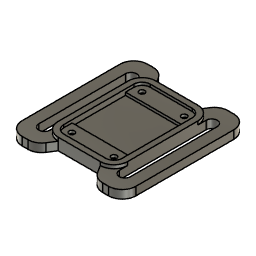
SquidSlimeCaseAUX (Autodesk Fusion 360 design; units mm, degrees)
Autodesk Fusion 360 part; units mm, degrees
note: some values were not read from the file. Set by a fixed rule: which face or edge a step refers to.
sketch "スケッチ1" plane through (0, 0, 0) normal (0, 0, 1) x (1, 0, 0)
  line L0 (52.54, 69.52) -> (67.78, 69.52)
  line L1 (70.32, 72.06) -> (70.32, 97.46)
  line L2 (67.78, 100) -> (52.54, 100)
  line L3 (50, 97.46) -> (50, 72.06)
  arc A0 (52.54, 100) -> (50, 97.46) centre (52.54, 97.46) ccw
  arc A1 (70.32, 97.46) -> (67.78, 100) centre (67.78, 97.46) ccw
  arc A2 (67.78, 69.52) -> (70.32, 72.06) centre (67.78, 72.06) ccw
  arc A3 (50, 72.06) -> (52.54, 69.52) centre (52.54, 72.06) ccw
  circle A4 centre (52.54, 97.46) radius 1
  circle A5 centre (67.78, 97.46) radius 1
  circle A6 centre (67.78, 72.06) radius 1
  circle A7 centre (52.54, 72.06) radius 1
  line L4 (60.16, 92.4) -> (60.16, 77.12)
  line L5 (65.24, 92.4) -> (55.08, 92.4)
  line L6 (55.08, 77.12) -> (65.24, 77.12)
  line L7 (55.08, 100) -> (55.08, 92.4)
  line L8 (55.08, 77.12) -> (55.08, 69.52)
  line L9 (65.24, 100) -> (65.24, 92.4)
  line L10 (65.24, 77.12) -> (65.24, 69.52)
  dimension "d7" = 2.54
  dimension "d8" = 2
  dimension "d9" = 2
  dimension "d10" = 2
  dimension "d11" = 2
  constraint horizontal L0
  constraint vertical L1
  constraint horizontal L2
  constraint vertical L3
  constraint tangent L2 A0
  constraint tangent L3 A0
  constraint tangent L1 A1
  constraint tangent L2 A1
  constraint equal A0 A1
  constraint tangent L0 A2
  constraint tangent L1 A2
  constraint equal A0 A2
  constraint tangent L3 A3
  constraint tangent L0 A3
  constraint equal A0 A3
  constraint concentric A0 A4
  constraint concentric A1 A5
  constraint concentric A2 A6
  constraint concentric A3 A7
  constraint coincident L6.start L7
  constraint collinear L7 L8
  constraint coincident L6 L4.end
  constraint coincident L6.end L9
  constraint collinear L9 L10
  constraint coincident L5 L4.start
  measures "d7" radius of A0
  measures "d8" diameter of A4
  measures "d9" diameter of A5
  measures "d10" diameter of A6
  measures "d11" diameter of A7
extrude "押し出し1" add sketch "スケッチ1" along normal blind 4.8 contours L0 L6 L8 L10 | L2 L5 L7 L9 makes body 1 at (61.8533, 94.9333, 0) makes body 2 at (58.4667, 72.0533, 0)
extrude "押し出し2" add 1 faces at (58.4667, 69.52, 3.2) along direction (0, -1, 0) blind 0.1 on bodies 2 bodies 2
extrude "押し出し3" add 1 faces at (61.8533, 100, 3.2) along direction (0, 1, 0) blind 0.1 on bodies 1 bodies 1
extrude "押し出し4" add sketch "スケッチ1" against normal blind 1 separate body makes body 3
combine "結合1" operation add target body 3 tool bodies 1 2
sketch "スケッチ2" plane through (0, 0, -1) normal (0, 0, -1) x (1, 0, 0)
  circle A0 centre (67.78, -72.06) radius 1
  circle A1 centre (52.54, -72.06) radius 1
  circle A2 centre (67.78, -97.46) radius 1
  circle A3 centre (52.54, -97.46) radius 1
  arc A4 (52.54, -69.52) -> (50, -72.06) centre (52.54, -72.06) ccw
  line L0 (50, -72.06) -> (50, -97.46)
  arc A5 (50, -97.46) -> (52.54, -100) centre (52.54, -97.46) ccw
  line L1 (52.54, -100) -> (67.78, -100)
  arc A6 (67.78, -100) -> (70.32, -97.46) centre (67.78, -97.46) ccw
  line L2 (70.32, -97.46) -> (70.32, -72.06)
  arc A7 (70.32, -72.06) -> (67.78, -69.52) centre (67.78, -72.06) ccw
  line L3 (67.78, -69.52) -> (52.54, -69.52)
  line L4 (52.54, -100.4) -> (67.78, -100.4)
  arc A8 (67.78, -100.4) -> (70.72, -97.46) centre (67.78, -97.46) ccw
  line L5 (70.72, -97.46) -> (70.72, -72.06)
  arc A9 (70.72, -72.06) -> (67.78, -69.12) centre (67.78, -72.06) ccw
  line L6 (67.78, -69.12) -> (52.54, -69.12)
  arc A10 (52.54, -69.12) -> (49.6, -72.06) centre (52.54, -72.06) ccw
  line L7 (49.6, -72.06) -> (49.6, -97.46)
  arc A11 (49.6, -97.46) -> (52.54, -100.4) centre (52.54, -97.46) ccw
  line L8 (52.54, -102.4) -> (67.78, -102.4)
  arc A12 (67.78, -102.4) -> (72.72, -97.46) centre (67.78, -97.46) ccw
  line L9 (72.72, -97.46) -> (72.72, -72.06)
  arc A13 (72.72, -72.06) -> (67.78, -67.12) centre (67.78, -72.06) ccw
  line L10 (67.78, -67.12) -> (52.54, -67.12)
  arc A14 (52.54, -67.12) -> (47.6, -72.06) centre (52.54, -72.06) ccw
  line L11 (47.6, -72.06) -> (47.6, -97.46)
  arc A15 (47.6, -97.46) -> (52.54, -102.4) centre (52.54, -97.46) ccw
  line L12 (60.16, -67.12) -> (60.16, -102.4)
  line L13 (55.08, -67.12) -> (55.08, -102.4)
  line L14 (65.24, -67.12) -> (65.24, -102.4)
  dimension "d24" = 0.4
  dimension "d25" = 2.4
  dimension "d58" = 5.08
  dimension "d59" = -5.08
  constraint midpoint L10 L12.start
  constraint midpoint L8 L12.end
extrude "押し出し5" add sketch "スケッチ2" against normal blind 1 separate body contours L6 L10 L12 L13 | L4 L6 A10 L7 A11 L8 L10 A14 L11 A15 L13 | L6 L10 L12 L14 | L4 L8 L12 L13 | L4 A8 L5 A9 L6 L8 A12 L9 A13 L10 L14 | L4 L8 L12 L14 makes body 4
extrude "押し出し6" add sketch "スケッチ2" along normal blind 1 bodies 4
extrude "押し出し7" add sketch "スケッチ2" along normal blind 1 contours A0 | A1 | A2 | A3 bodies 4
extrude "押し出し8" add sketch "スケッチ2" against normal blind 8 separate body contours A0 | A1 | A2 | A3 | A4 L0 A5 L1 L3 L13 | A4 L0 A5 L1 L3 L4 L6 A10 L7 A11 L13 | L3 L6 L12 L13 | L1 L3 L12 L13 | L3 L6 L12 L14 | L1 L3 L12 L14 | L6 L10 L12 L13 | L4 L6 A10 L7 A11 L8 L10 A14 L11 A15 L13 | L1 L4 L12 L13 | L1 A6 L2 A7 L3 L4 A8 L5 A9 L6 L14 | L1 A6 L2 A7 L3 L14 | L6 L10 L12 L14 | L1 L4 L12 L14 | L4 L8 L12 L13 | L4 A8 L5 A9 L6 L8 A12 L9 A13 L10 L14 | L4 L8 L12 L14 makes body 5
extrude "押し出し9" cut 1 faces at (64.3467, 88.9933, -1) along direction (0, 0, 1) blind 1 on bodies 5 bodies 5
extrude "押し出し10" cut 2 faces at (61.8533, 94.9667, 4.8) (58.4667, 71.9867, 4.8) along direction (0, 0, 1) blind 7 on bodies 3 bodies 5
extrude "押し出し11" cut 1 faces at (58.4667, 69.42, 5.5333) along direction (0, -1, 0) blind 10 on bodies 5 bodies 5
extrude "押し出し12" cut 1 faces at (61.8533, 100.1, 5.5333) along direction (0, 1, 0) blind 11 on bodies 5 bodies 5
extrude "押し出し13" cut 1 faces at (61.8533, 100.1, 3.2) along direction (0, 1, 0) blind 8 on bodies 3 bodies 5
extrude "押し出し14" cut 1 faces at (58.4667, 69.42, 3.2) along direction (0, -1, 0) blind 9 on bodies 3 bodies 5
extrude "押し出し15" cut sketch "スケッチ2" against normal blind 5.8 contours A0 | A1 | A2 | A3 | A4 L0 A5 L1 L3 L13 | A4 L0 A5 L1 L3 L4 L6 A10 L7 A11 L13 | L3 L6 L12 L13 | L1 L3 L12 L13 | L3 L6 L12 L14 | L1 L3 L12 L14 | L1 L4 L12 L13 | L1 A6 L2 A7 L3 L4 A8 L5 A9 L6 L14 | L1 A6 L2 A7 L3 L14 | L1 L4 L12 L14 bodies 5
extrude "押し出し16" cut 2 faces at (65.24, 98.4, 6.2667) (65.24, 71.12, 6.2667) along direction (1, 0, 0) blind 0.25 on bodies 5 bodies 5
extrude "押し出し17" cut 2 faces at (55.08, 71.12, 6.2667) (55.08, 98.4, 6.2667) along direction (-1, 0, 0) blind 0.25 on bodies 5 bodies 5
extrude "押し出し18" cut 1 faces at (61.9367, 92.4, 6.2667) along direction (0, -1, 0) blind 0.25 on bodies 5 bodies 5
extrude "押し出し19" cut 1 faces at (61.9367, 77.12, 5.5333) along direction (0, 1, 0) blind 0.25 on bodies 5 bodies 5
extrude "押し出し20" cut sketch "スケッチ1" against normal blind 12 contours A4 | A5 | A6 | A7 bodies 4
extrude "押し出し21" add sketch "スケッチ2" against normal blind 5.8 contours A4 L0 A5 L1 L3 L13 | A4 L0 A5 L1 L3 L4 L6 A10 L7 A11 L13 | L1 A6 L2 A7 L3 L4 A8 L5 A9 L6 L14 | L1 A6 L2 A7 L3 L14 bodies 5
extrude "押し出し22" cut 2 faces at (69.8618, 88.683, -1) (50.4582, 88.683, -1) along direction (0, 0, 1) blind 1 on bodies 5 bodies 5
extrude "押し出し23" cut 1 faces at (65.24, 82.2967, 1.6) along direction (1, 0, 0) blind 0.25 on bodies 5 bodies 5
extrude "押し出し24" cut 1 faces at (55.08, 82.2967, 1.6) along direction (-1, 0, 0) blind 0.25 on bodies 5 bodies 5
extrude "押し出し25" cut 1 faces at (58.3833, 87.2233, 7) along direction (0, 0, -1) blind 0.2 on bodies 5 bodies 5
extrude "押し出し26" add 1 faces at (57.7867, 88.7047, -2) along direction (0, 0, -1) blind 1.5 separate body on bodies 4 makes body 6
move_face "面をオフセット1" offset -0.75 4 faces at (51.8783, 71.3102, -3) (53.5091, 97.7068, -3) (67.014, 96.8172, -3) (68.7491, 72.3068, -3) on bodies 6
combine "結合2" operation add target body 4 tool bodies 6
extrude "押し出し27" add 1 faces at (57.9117, 88.4882, -3.5) along direction (0, 0, -1) blind 0.5 on bodies 4 bodies 4
sketch "スケッチ3" plane through (0, 0, -4) normal (0, 0, -1) x (1, 0, 0)
  circle A0 centre (52.54, -97.46) radius 1.75
  circle A1 centre (52.54, -72.06) radius 1.75
  circle A2 centre (67.78, -97.46) radius 1.75
  circle A3 centre (67.78, -72.06) radius 1.75
  arc A4 (47.6, -97.46) -> (52.54, -102.4) centre (52.54, -97.46) ccw
  line L0 (52.54, -102.4) -> (67.78, -102.4)
  arc A5 (67.78, -102.4) -> (72.72, -97.46) centre (67.78, -97.46) ccw
  line L1 (72.72, -97.46) -> (72.72, -72.06)
  arc A6 (72.72, -72.06) -> (67.78, -67.12) centre (67.78, -72.06) ccw
  line L2 (67.78, -67.12) -> (52.54, -67.12)
  arc A7 (52.54, -67.12) -> (47.6, -72.06) centre (52.54, -72.06) ccw
  line L3 (47.6, -72.06) -> (47.6, -97.46)
  line L4 (76.72, -97.46) -> (76.72, -74.06)
  line L5 (80.72, -97.46) -> (80.72, -72.06)
  line L6 (43.6, -74.06) -> (43.6, -97.46)
  line L7 (39.6, -72.06) -> (39.6, -97.46)
  line L8 (60.16, -67.12) -> (60.16, -102.4)
  arc A8 (80.72, -72.06) -> (75.78, -67.12) centre (75.78, -72.06) ccw
  arc A9 (44.54, -67.12) -> (39.6, -72.06) centre (44.54, -72.06) ccw
  line L9 (44.54, -67.12) -> (75.78, -67.12)
  line L10 (47.6, -84.76) -> (72.72, -84.76)
  line L11 (47.6, -74.06) -> (47.6, -97.46)
  line L12 (72.72, -74.06) -> (72.72, -97.46)
  arc A10 (45.6, -72.06) -> (43.6, -74.06) centre (45.6, -74.06) ccw
  arc A11 (47.6, -74.06) -> (45.6, -72.06) centre (45.6, -74.06) ccw
  arc A12 (74.72, -72.06) -> (72.72, -74.06) centre (74.72, -74.06) ccw
  arc A13 (76.72, -74.06) -> (74.72, -72.06) centre (74.72, -74.06) ccw
  arc A14 (75.78, -102.4) -> (80.72, -97.46) centre (75.78, -97.46) ccw
  arc A15 (74.72, -97.46) -> (76.72, -95.46) centre (74.72, -95.46) ccw
  arc A16 (72.72, -95.46) -> (74.72, -97.46) centre (74.72, -95.46) ccw
  line L13 (44.54, -102.4) -> (75.78, -102.4)
  arc A17 (39.6, -97.46) -> (44.54, -102.4) centre (44.54, -97.46) ccw
  arc A18 (43.6, -95.46) -> (45.6, -97.46) centre (45.6, -95.46) ccw
  arc A19 (45.6, -97.46) -> (47.6, -95.46) centre (45.6, -95.46) ccw
  dimension "d76" = 8
  dimension "d78" = 8
  dimension "d79" = 2
  constraint midpoint L2 L8.start
  constraint midpoint L0 L8.end
  constraint symmetric L8 L5.end L7.start
  constraint symmetric L8 A8.end A9.start
  constraint symmetric L8 A8 A9
  constraint tangent A8 L9
  constraint midpoint L3 L10.start
  constraint midpoint L1 L10.end
  constraint coincident A4.start L3.end
  constraint coincident A5.end L1.start
  constraint tangent L6 A10
  constraint tangent L11 A11
  constraint equal A10 A11
  constraint coincident A10.start A11.end
  constraint tangent L12 A12
  constraint equal A10 A12
  constraint tangent L4 A13
  constraint equal A10 A13
  constraint coincident A12.start A13.end
  constraint symmetric L5.end L10 L5.start
  constraint symmetric A8.end L10 A14.start
  constraint symmetric A8 L10 A14
  constraint symmetric L7.start L10 L7.end
  constraint symmetric A9.start L10 L13.start
  constraint symmetric A9 L10 A17
  constraint symmetric L10 L6.start A18.start
  constraint symmetric L10 A10.start A18.end
  constraint symmetric L10 A10 A18
  constraint symmetric L10 L11.start A19.end
  constraint symmetric L10 A11 A19
  constraint symmetric L10 A12.start A15.start
  constraint symmetric L10 L12.start A16.start
  constraint symmetric L10 A12 A16
  constraint symmetric L10 L4.end A15.end
  constraint symmetric L10 A13 A15
  measures "d79" radius of A10
extrude "押し出し28" add sketch "スケッチ3" against normal blind 4 separate body contours A4 A7 L3 L6 L7 A9 L9 L11 A10 A11 L13 A17 A18 A19 | A5 L1 A6 L4 L5 A8 L9 L12 A12 A13 A14 A15 A16 L13 makes body 7 at (40.9333, 81.1933, 0) makes body 8 at (79.3867, 88.3267, -4)
combine "結合3" operation add target body 4 tool bodies 7 8
extrude "押し出し29" cut sketch "スケッチ3" against normal blind 12 contours A4 A7 L3 L6 L7 A9 L9 L11 A10 A11 L13 A17 A18 A19 | A5 L1 A6 L4 L5 A8 L9 L12 A12 A13 A14 A15 A16 L13 bodies 4
extrude "押し出し30" add sketch "スケッチ3" against normal blind 3 contours A4 A7 L3 L6 L7 A9 L9 L11 A10 A11 L13 A17 A18 A19 | A5 L1 A6 L4 L5 A8 L9 L12 A12 A13 A14 A15 A16 L13 bodies 4
copy_body "ボディのコピーと貼り付け1" bodies 4 makes body 9
extrude "押し出し31" cut 2 faces at (40.9333, 81.1933, -1) (79.3867, 88.3267, -1) along direction (0, 0, -1) blind 12 on bodies 9 bodies 9
sketch "スケッチ4" plane through (0, 0, -4) normal (0, 0, -1) x (1, 0, 0)
  arc A0 (75.78, -117.4) -> (80.72, -112.46) centre (75.78, -112.46) ccw
  arc A1 (74.72, -112.46) -> (76.72, -110.46) centre (74.72, -110.46) ccw
  arc A2 (72.72, -110.46) -> (74.72, -112.46) centre (74.72, -110.46) ccw
  arc A3 (68.72, -112.46) -> (73.66, -117.4) centre (73.66, -112.46) ccw
  line L0 (75.78, -117.4) -> (73.66, -117.4)
  line L1 (47.6, -84.76) -> (72.72, -84.76)
  arc A4 (80.72, -57.06) -> (75.78, -52.12) centre (75.78, -57.06) ccw
  arc A5 (73.66, -52.12) -> (68.72, -57.06) centre (73.66, -57.06) ccw
  arc A6 (76.72, -59.06) -> (74.72, -57.06) centre (74.72, -59.06) ccw
  line L2 (75.78, -52.12) -> (73.66, -52.12)
  arc A7 (74.72, -57.06) -> (72.72, -59.06) centre (74.72, -59.06) ccw
  line L3 (80.72, -112.46) -> (80.72, -57.06)
  arc A8 (72.72, -72.06) -> (67.78, -67.12) centre (67.78, -72.06) ccw
  line L4 (68.72, -57.06) -> (67.78, -67.12)
  arc A9 (67.78, -102.4) -> (72.72, -97.46) centre (67.78, -97.46) ccw
  line L5 (68.72, -112.46) -> (67.78, -102.4)
  line L6 (76.72, -59.06) -> (76.72, -110.46)
  line L7 (72.72, -59.06) -> (72.72, -110.46)
  line L8 (60.16, -67.12) -> (60.16, -102.4)
  line L9 (43.6, -59.06) -> (43.6, -110.46)
  arc A10 (46.66, -117.4) -> (51.6, -112.46) centre (46.66, -112.46) ccw
  line L10 (44.54, -117.4) -> (46.66, -117.4)
  arc A11 (45.6, -112.46) -> (47.6, -110.46) centre (45.6, -110.46) ccw
  arc A12 (43.6, -110.46) -> (45.6, -112.46) centre (45.6, -110.46) ccw
  line L11 (47.6, -59.06) -> (47.6, -110.46)
  arc A13 (45.6, -57.06) -> (43.6, -59.06) centre (45.6, -59.06) ccw
  line L12 (39.6, -112.46) -> (39.6, -57.06)
  arc A14 (52.54, -67.12) -> (47.6, -72.06) centre (52.54, -72.06) ccw
  line L13 (51.6, -57.06) -> (52.54, -67.12)
  arc A15 (39.6, -112.46) -> (44.54, -117.4) centre (44.54, -112.46) ccw
  arc A16 (47.6, -97.46) -> (52.54, -102.4) centre (52.54, -97.46) ccw
  arc A17 (47.6, -59.06) -> (45.6, -57.06) centre (45.6, -59.06) ccw
  arc A18 (44.54, -52.12) -> (39.6, -57.06) centre (44.54, -57.06) ccw
  line L14 (44.54, -52.12) -> (46.66, -52.12)
  arc A19 (51.6, -57.06) -> (46.66, -52.12) centre (46.66, -57.06) ccw
  line L15 (51.6, -112.46) -> (52.54, -102.4)
  point P0 (47.6, -84.76)
  constraint tangent A3 L0
  constraint symmetric A0.start L1 A4.end
  constraint symmetric A0.end L1 A4.start
  constraint symmetric A0 L1 A4
  constraint symmetric A2.start L1 A7.end
  constraint symmetric A1.start L1 A6.end
  constraint symmetric A1.end L1 A6.start
  constraint symmetric A1 L1 A6
  constraint symmetric A2 L1 A7
  constraint symmetric A3.end L1 A5.start
  constraint symmetric A3.start L1 A5.end
  constraint symmetric A3 L1 A5
  constraint tangent A4 L3
  constraint symmetric L1 A5.end A3.start
  constraint symmetric L1 A8.start A9.end
  constraint symmetric L1 A8.end A9.start
  constraint symmetric L1 A8 A9
  constraint tangent A1 L6
  constraint tangent A2 L7
  constraint symmetric A0.start L8 L10.start
  constraint symmetric A0.end L8 L12.start
  constraint symmetric A0 L8 A15
  constraint symmetric A2.start L8 A11.end
  constraint symmetric A1.start L8 A11.start
  constraint symmetric A1.end L8 L9.end
  constraint symmetric A1 L8 A12
  constraint symmetric A2 L8 A11
  constraint symmetric A3.end L8 A10.start
  constraint symmetric A3.start L8 A10.end
  constraint symmetric A3 L8 A10
  constraint symmetric L1.end L8 P0
  constraint symmetric A7.end L8 L11.start
  constraint symmetric A6.start L8 L9.start
  constraint symmetric A5.start L8 L14.end
  constraint symmetric A4.start L8 L12.end
  constraint symmetric A4.end L8 A18.start
  constraint symmetric A6.end L8 A13.start
  constraint symmetric A5.end L8 L13.start
  constraint symmetric A4 L8 A18
  constraint symmetric A5 L8 A19
  constraint symmetric A6 L8 A13
  constraint symmetric A7 L8 A17
  constraint symmetric A8.start L8 A14.end
  constraint symmetric A8.end L8 A14.start
  constraint symmetric A8 L8 A14
  constraint symmetric A9.end L8 A16.start
  constraint symmetric A9.start L8 A16.end
  constraint symmetric A9 L8 A16
extrude "押し出し32" add sketch "スケッチ4" against normal blind 3 contours A0 A1 A2 A3 L0 A4 A5 A6 L2 A7 L3 A8 L4 A9 L5 L6 L7 | L9 A10 L10 A11 A12 L11 A13 L12 A14 L13 A15 A16 A17 A18 L14 A19 L15 bodies 9
sketch "スケッチ5" plane through (0, 0, -1) normal (0, 0, 1) x (-1, 0, 0)
  circle A0 centre (-52.54, -97.46) radius 1
  circle A1 centre (-52.54, -72.06) radius 1
  circle A2 centre (-67.78, -97.46) radius 1
  circle A3 centre (-67.78, -72.06) radius 1
  line L0 (-49.6, -97.46) -> (-49.6, -72.06)
  arc A4 (-49.6, -72.06) -> (-52.54, -69.12) centre (-52.54, -72.06) ccw
  line L1 (-52.54, -69.12) -> (-67.78, -69.12)
  arc A5 (-67.78, -69.12) -> (-70.72, -72.06) centre (-67.78, -72.06) ccw
  line L2 (-70.72, -72.06) -> (-70.72, -97.46)
  arc A6 (-70.72, -97.46) -> (-67.78, -100.4) centre (-67.78, -97.46) ccw
  line L3 (-67.78, -100.4) -> (-52.54, -100.4)
  arc A7 (-52.54, -100.4) -> (-49.6, -97.46) centre (-52.54, -97.46) ccw
  line L4 (-60.16, -75.12) -> (-49.6, -75.12)
  line L5 (-60.16, -75.12) -> (-70.72, -75.12)
  line L6 (-49.6, -84.76) -> (-70.72, -84.76)
  line L7 (-60.16, -94.4) -> (-49.6, -94.4)
  line L8 (-60.16, -94.4) -> (-70.72, -94.4)
  constraint coincident L0 L4.end
  constraint perpendicular L0 L4
  constraint perpendicular L2 L5
  constraint midpoint L0 L6.start
  constraint midpoint L2 L6.end
  constraint symmetric L4.start L6 L7.start
  constraint symmetric L4.end L6 L7.end
  constraint symmetric L5.end L6 L8.end
extrude "押し出し33" cut sketch "スケッチ5" against normal blind 1 contours L0 L2 L6 L7 L8 | L0 L2 L4 L5 L6 bodies 4 9
sketch "スケッチ6" plane through (0, 0, -4) normal (0, 0, -1) x (1, 0, 0)
  arc A0 (80.72, -67.06) -> (75.78, -62.12) centre (75.78, -67.06) ccw
  line L0 (75.78, -62.12) -> (73.66, -62.12)
  arc A1 (73.66, -62.12) -> (69.4828, -64.4228) centre (73.66, -67.06) ccw
  arc A2 (72.72, -72.06) -> (67.78, -67.12) centre (67.78, -72.06) ccw
  arc A3 (72.72, -72.06) -> (67.78, -67.12) centre (67.78, -72.06) ccw
  line L1 (67.78, -67.12) -> (69.4828, -64.4228)
  arc A4 (76.72, -69.06) -> (74.72, -67.06) centre (74.72, -69.06) ccw
  arc A5 (74.72, -67.06) -> (72.72, -69.06) centre (74.72, -69.06) ccw
  line L2 (47.6, -84.76) -> (72.72, -84.76)
  arc A6 (72.72, -100.46) -> (74.72, -102.46) centre (74.72, -100.46) ccw
  arc A7 (74.72, -102.46) -> (76.72, -100.46) centre (74.72, -100.46) ccw
  arc A8 (75.78, -107.4) -> (80.72, -102.46) centre (75.78, -102.46) ccw
  line L3 (75.78, -107.4) -> (73.66, -107.4)
  arc A9 (69.4828, -105.0972) -> (73.66, -107.4) centre (73.66, -102.46) ccw
  line L4 (67.78, -102.4) -> (69.4828, -105.0972)
  arc A10 (67.78, -102.4) -> (72.72, -97.46) centre (67.78, -97.46) ccw
  line L5 (72.72, -100.46) -> (72.72, -69.06)
  line L6 (76.72, -69.06) -> (76.72, -100.46)
  line L7 (80.72, -102.46) -> (80.72, -67.06)
  line L8 (60.16, -67.12) -> (60.16, -102.4)
  line L9 (47.6, -100.46) -> (47.6, -69.06)
  arc A11 (46.66, -107.4) -> (50.8372, -105.0972) centre (46.66, -102.46) ccw
  line L10 (39.6, -102.46) -> (39.6, -67.06)
  arc A12 (43.6, -100.46) -> (45.6, -102.46) centre (45.6, -100.46) ccw
  arc A13 (52.54, -67.12) -> (47.6, -72.06) centre (52.54, -72.06) ccw
  line L11 (52.54, -102.4) -> (50.8372, -105.0972)
  line L12 (44.54, -107.4) -> (46.66, -107.4)
  arc A14 (45.6, -102.46) -> (47.6, -100.46) centre (45.6, -100.46) ccw
  line L13 (43.6, -69.06) -> (43.6, -100.46)
  arc A15 (47.6, -97.46) -> (52.54, -102.4) centre (52.54, -97.46) ccw
  line L14 (52.54, -67.12) -> (50.8372, -64.4228)
  arc A16 (39.6, -102.46) -> (44.54, -107.4) centre (44.54, -102.46) ccw
  arc A17 (52.54, -67.12) -> (47.6, -72.06) centre (52.54, -72.06) ccw
  arc A18 (47.6, -69.06) -> (45.6, -67.06) centre (45.6, -69.06) ccw
  line L15 (44.54, -62.12) -> (46.66, -62.12)
  arc A19 (44.54, -62.12) -> (39.6, -67.06) centre (44.54, -67.06) ccw
  arc A20 (50.8372, -64.4228) -> (46.66, -62.12) centre (46.66, -67.06) ccw
  arc A21 (45.6, -67.06) -> (43.6, -69.06) centre (45.6, -69.06) ccw
  point P0 (47.6, -84.76)
  constraint tangent A1 L1
  constraint symmetric A0.start L2 A8.end
  constraint symmetric A0.end L2 A8.start
  constraint symmetric L0.end L2 L3.end
  constraint symmetric A0 L2 A8
  constraint symmetric A1 L2 A9
  constraint symmetric A2.start L2 A10.end
  constraint symmetric A2.end L2 L4.start
  constraint symmetric A3 L2 A10
  constraint symmetric A1.end L2 A9.start
  constraint symmetric A4.end L2 A6.end
  constraint symmetric A5.end L2 A6.start
  constraint symmetric A4.start L2 A7.end
  constraint symmetric A4 L2 A7
  constraint symmetric A5 L2 A6
  constraint tangent A5 L5
  constraint tangent A7 L6
  constraint tangent A0 L7
  constraint symmetric A0.start L8 L10.end
  constraint symmetric A0.end L8 L15.start
  constraint symmetric L0.end L8 L15.end
  constraint symmetric A0 L8 A19
  constraint symmetric A1 L8 A20
  constraint symmetric A2.start L8 A13.end
  constraint symmetric A2.end L8 A13.start
  constraint symmetric A2 L8 A13
  constraint symmetric A3 L8 A17
  constraint symmetric A1.end L8 L14.end
  constraint symmetric A4.end L8 A18.end
  constraint symmetric A5.end L8 L9.end
  constraint symmetric A4.start L8 L13.start
  constraint symmetric A4 L8 A21
  constraint symmetric A5 L8 A18
  constraint symmetric L2.end L8 P0
  constraint symmetric A6.end L8 A12.end
  constraint symmetric A6.start L8 L9.start
  constraint symmetric A6 L8 A14
  constraint symmetric A7.end L8 A12.start
  constraint symmetric A7 L8 A12
  constraint symmetric A8.end L8 L10.start
  constraint symmetric A8.start L8 L12.start
  constraint symmetric A8 L8 A16
  constraint symmetric L3.end L8 A11.start
  constraint symmetric A9.start L8 A11.end
  constraint symmetric A9 L8 A11
  constraint symmetric L4.start L8 L11.start
  constraint symmetric A10.end L8 A15.start
  constraint symmetric A10 L8 A15
copy_body "ボディのコピーと貼り付け2" bodies 4 makes body 10
extrude "押し出し34" cut 2 faces at (40.9333, 81.1933, -1) (79.3867, 88.3267, -1) along direction (0, 0, -1) blind 14 on bodies 10 bodies 10
extrude "押し出し35" add sketch "スケッチ6" against normal blind 3 contours A0 L0 A1 A2 A3 L1 A4 A5 A6 A7 A8 L3 A9 L4 A10 L5 L6 L7 | L9 A11 L10 A12 A13 L11 L12 A14 L13 A15 L14 A16 A17 A18 L15 A19 A20 A21 bodies 10
fillet "フィレット1" radius 5 4 edges at (52.54, 102.4, -2.5) (67.78, 102.4, -2.5) (67.78, 67.12, -2.5) (52.54, 67.12, -2.5) on bodies 9
sketch "スケッチ7" plane through (0, 0, 0) normal (0, 0, -1) x (1, 0, 0)
  line L0 (54.83, -102.4) -> (54.83, -67.12)
  line L1 (54.83, -67.12) -> (52.54, -67.12)
  arc A0 (52.54, -67.12) -> (47.6, -72.06) centre (52.54, -72.06) ccw
  line L2 (47.6, -72.06) -> (47.6, -97.46)
  arc A1 (47.6, -97.46) -> (52.54, -102.4) centre (52.54, -97.46) ccw
  line L3 (52.54, -102.4) -> (54.83, -102.4)
  circle A2 centre (52.54, -72.06) radius 1
  circle A3 centre (52.54, -97.46) radius 1
  line L4 (54.83, -102.4) -> (54.83, -94.9)
  line L5 (54.83, -67.12) -> (54.83, -74.62)
  line L6 (54.83, -74.62) -> (42, -74.62)
  line L7 (54.83, -94.9) -> (43, -94.9)
  dimension "d99" = 7.5
  dimension "d100" = 7.5
  constraint coincident L0.start L3.end
  constraint perpendicular L3 L4
  constraint coincident L0.end L1.start
  constraint perpendicular L1 L5
  constraint perpendicular L0 L6
  constraint perpendicular L4 L7
  measures "d99" distance of L0.start L4.end
  measures "d100" distance of L0.end L5.end
extrude "押し出し36" cut sketch "スケッチ7" against normal blind 4.8 contours L0 L2 L6 L7 bodies 5
sketch "スケッチ8" plane through (0, 0, 0) normal (0, 0, -1) x (1, 0, 0)
  line L0 (65.49, -67.12) -> (65.49, -102.4)
  line L1 (65.49, -102.4) -> (67.78, -102.4)
  arc A0 (67.78, -102.4) -> (72.72, -97.46) centre (67.78, -97.46) ccw
  line L2 (72.72, -97.46) -> (72.72, -72.06)
  arc A1 (72.72, -72.06) -> (67.78, -67.12) centre (67.78, -72.06) ccw
  line L3 (67.78, -67.12) -> (65.49, -67.12)
  circle A2 centre (67.78, -72.06) radius 1
  circle A3 centre (67.78, -97.46) radius 1
  line L4 (65.49, -102.4) -> (65.49, -94.9)
  line L5 (65.49, -67.12) -> (65.49, -74.62)
  line L6 (65.49, -94.9) -> (81, -94.9)
  line L7 (65.49, -74.62) -> (81, -74.62)
  dimension "d103" = 7.5
  dimension "d104" = 7.5
  constraint coincident L0.end L1.start
  constraint perpendicular L1 L4
  constraint coincident L0.start L3.end
  constraint perpendicular L3 L5
  constraint perpendicular L2 L6
  constraint perpendicular L2 L7
  measures "d103" distance of L0.end L4.end
  measures "d104" distance of L0.start L5.end
extrude "押し出し37" cut sketch "スケッチ8" against normal blind 4.8 contours L0 L2 L6 L7 bodies 5
extrude "押し出し38" add sketch "スケッチ7" sketch "スケッチ8" against normal blind 4.8 separate body contours L0 L2 L6 L7 of sketch 2 contours L0 L2 L6 L7 makes body 11 at (50.01, 88.14, 0) makes body 12 at (67.9, 81.38, 0)
extrude "押し出し39" cut 1 faces at (54.83, 81.38, 3.2) along direction (-1, 0, 0) blind 6.23 on bodies 11 bodies 11
extrude "押し出し40" cut 1 faces at (65.49, 88.14, 3.2) along direction (1, 0, 0) blind 6.23 on bodies 12 bodies 12
combine "結合4" operation add target body 5 tool bodies 11 12
extrude "押し出し41" add 1 faces at (71.72, 88.14, 3.2) along direction (-1, 0, 0) blind 1 on bodies 5 bodies 5
extrude "押し出し42" add 1 faces at (48.6, 81.38, 3.2) along direction (1, 0, 0) blind 1 on bodies 5 bodies 5
extrude "押し出し43" add 2 faces at (72.0533, 81.38, 0) (48.2667, 81.38, 0) along direction (0, 0, -1) blind 1.5 on bodies 5 bodies 5
move_face "面をオフセット2" offset 0.075 8 faces at (68.7491, 71.8132, -1) (68.7491, 71.8132, 3.2) (53.5388, 72.0102, -0.5) (53.5388, 72.0102, 1.6) (53.5091, 97.2132, -1) (53.5091, 97.2132, 3.2) (67.014, 98.1028, -1) (67.014, 98.1028, 3.2) on bodies 5
extrude "押し出し44" add 1 faces at (57.9117, 88.4882, -4) along direction (0, 0, -1) blind 1 on bodies 9 bodies 9
extrude "押し出し45" cut 2 faces at (40.9333, 76.1933, -1) (79.3867, 93.3267, -1) along direction (0, 0, -1) blind 1 on bodies 9 bodies 9
extrude "押し出し46" cut 2 faces at (40.9333, 81.1933, -1) (79.3867, 88.3267, -1) along direction (0, 0, -1) blind 0.75 on bodies 4 bodies 4
extrude "押し出し47" add 1 faces at (57.9117, 88.4882, -4) along direction (0, 0, -1) blind 0.75 on bodies 4 bodies 4
move_face "面をオフセット4" offset -0.5 4 faces at (69.4759, 97.8918, -3.8333) (50.9274, 96.7802, -3.8333) (54.1526, 72.7398, -3.8333) (66.1674, 71.3802, -3.8333) on bodies 4
move_face "面をオフセット5" offset -0.125 4 faces at (51.8418, 71.3441, -1.6667) (67.014, 96.8172, -1.6667) (53.5091, 97.7068, -1.6667) (68.7491, 72.3068, -1.6667) on bodies 4
move_face "面をオフセット6" offset -0.125 4 faces at (67.014, 96.8172, -1.6667) (53.5091, 97.7068, -1.6667) (51.8418, 71.3441, -1.6667) (68.7491, 72.3068, -1.6667) on bodies 9
extrude "押し出し48" add 1 faces at (62.4083, 88.4882, -4) along direction (0, 0, -1) blind 0.25 on bodies 10 bodies 10
extrude "押し出し49" cut 2 faces at (40.9333, 89.9933, -1) (79.3867, 89.9933, -1) along direction (0, 0, -1) blind 0.25 on bodies 10 bodies 10
move_face "面をオフセット7" offset -0.5 4 faces at (54.1526, 72.7398, -3.5) (66.1355, 71.4615, -3.5) (50.8955, 96.8615, -3.5) (69.4759, 97.8918, -3.5) on bodies 10
hidden bodies 3 5 4 9
equation "d58 = ( 10.16 / 2 ) * 1 mm"
equation "d119 = ( 0.15 / 2 ) * 1 mm"
equation "d131 = ( -0.5 / 4 ) * 1 mm"
named bodies: "Mock", "SquidSlimeCaseAUXBottom", "SquidSlimeCaseAUXUpper", "SquidSlimeCaseAUXBottomLongVer", "SquidSlimeCaseAUXBottom (1)", "SquidSlimeCaseAUXBottomMidium"
